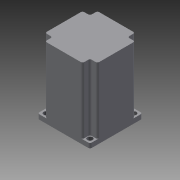
# Autodesk Inventor part: nema23_HS8630
Saved by Autodesk Inventor 2014 (Build 180170000, 170)
## iProperties
Created: 2014-08-18
Part Number: nema23_HS8630
Material: Generic
Document SubType Name: Modeling
Designer: Matthew
Density: 1 g/cm^3
Appearance: Default
Author: Matthew
Autodesk Inventor part; units mm, degrees
ref_plane "YZ Plane" through (0, 0, 0) normal (1, 0, 0) x (0, 1, 0)
ref_plane "XZ Plane" through (0, 0, 0) normal (0, 1, 0) x (-1, 0, 0)
ref_plane "XY Plane" through (0, 0, 0) normal (0, 0, 1) x (1, 0, 0)
sketch "Sketch1" plane through (0, 0, 0) normal (0, 0, 1) x (1, 0, 0)
  line L0 (-28.2, -28.2) -> (28.2, -28.2)
  line L1 (28.2, -28.2) -> (28.2, 28.2)
  line L2 (28.2, 28.2) -> (-28.2, 28.2)
  line L3 (-28.2, 28.2) -> (-28.2, -28.2)
  line L4 (-28.2, -28.2) -> (28.2, 28.2) construction
  line L5 (28.2, -28.2) -> (-28.2, 28.2) construction
  point P0 (0, 0)
  point P1 (-23.57, 23.57)
  point P2 (23.57, 23.57)
  point P3 (23.57, -23.57)
  point P4 (-23.57, -23.57)
  dimension "d0" = 56.4
  dimension "d1" = 56.4
  dimension "d2" = 47.14
  constraints: 12 end point, 4 point on line, 2 horizontal alignment, 2 midpoint, 2 parallel, 2 vertical alignment, 1 horizontal, 1 perpendicular
  measures "d0" distance of L2.end L1.end
  measures "d1" distance of L0.end L1.end
  measures "d2" distance of point (23.57, 23.57) point (-23.57, 23.57)
extrude "Extrusion1" add sketch "Sketch1" along normal blind 76
sketch "Sketch2" plane through (0, 0, 0) normal (0, 0, -1) x (-1, 0, 0)
  point P0 (0, 0)
  point P1 (-23.57, 23.57)
  point P2 (23.57, 23.57)
  point P3 (23.57, -23.57)
  point P4 (-23.57, -23.57)
  dimension "d5" = 47.14
  dimension "d6" = 47.14
  dimension "d8" = 23.57
  dimension "d9" = 23.57
  constraints: 2 horizontal alignment, 2 vertical alignment
  measures "d5" distance of point (23.57, 23.57) point (-23.57, 23.57)
  measures "d6" distance of point (23.57, -23.57) point (23.57, 23.57)
  measures "d8" horizontal distance of point (0, 0) point (-23.57, 23.57)
  measures "d9" horizontal distance of point (-23.57, -23.57) point (0, 0)
hole "Hole1" at (23.57, 23.57, 0) at (-23.57, 23.57, 0) at (-23.57, -23.57, 0) at (23.57, -23.57, 0) direction (0, 0, 1) diameter 5.5 depth 8 tip angle 118
thread "Thread1" size "M5x0.8" class "6H" standard "ANSI Metric M Profile" full length
thread "Thread2" size "M5.5x0.5" class "6H" standard "ANSI Metric M Profile" full length
thread "Thread3" size "M5.5x0.5" class "6H" standard "ANSI Metric M Profile" full length
thread "Thread4" size "M5.5x0.5" class "6H" standard "ANSI Metric M Profile" full length
sketch "Sketch3" plane through (0, 0, 0) normal (0, 0, -1) x (-1, 0, 0)
  circle A0 centre (0, 0) radius 19.05
  dimension "d25" = 38.1
  constraints: 1 centre point, 1 coincident
  measures "d25" diameter of A0
extrude "Extrusion2" add sketch "Sketch3" along normal blind 1.6
sketch "Sketch4" plane through (0, 0, -1.6) normal (0, 0, -1) x (-1, 0, 0)
  circle A0 centre (0, 0) radius 19.05 projected
  circle A1 centre (0, 0) radius 3.175
  dimension "d28" = 6.35
  constraints: 1 centre point, 1 coincident
  measures "d28" diameter of A1
extrude "Extrusion3" add sketch "Sketch4" along normal blind 21 contours A1
sketch "Sketch5" plane through (0, 0, 76) normal (0, 0, 1) x (1, 0, 0)
  line L0 (-28.2, -28.2) -> (28.2, -28.2) projected
  line L1 (28.2, -28.2) -> (28.2, 28.2) projected
  line L2 (28.2, 28.2) -> (-28.2, 28.2) projected
  line L3 (-28.2, 28.2) -> (-28.2, -28.2) projected
  line L4 (-28.2, 20.2) -> (-20.2, 20.2)
  line L5 (-20.2, 20.2) -> (-20.2, 28.2)
  line L6 (20.2, 28.2) -> (20.2, 20.2)
  line L7 (20.2, 20.2) -> (28.2, 20.2)
  line L8 (28.2, -20.2) -> (20.2, -20.2)
  line L9 (-20.2, -28.2) -> (-20.2, -20.2)
  line L10 (-20.2, -20.2) -> (-28.2, -20.2)
  line L11 (20.2, -20.2) -> (20.2, -28.2)
  line L12 (-20.2, 28.2) -> (20.2, 28.2)
  line L13 (28.2, 20.2) -> (28.2, -20.2)
  line L14 (-28.2, 20.2) -> (-28.2, -20.2)
  line L15 (-20.2, -28.2) -> (20.2, -28.2)
  point P0 (0, 0)
  dimension "d31" = 8
  dimension "d32" = 8
  dimension "d33" = 8
  dimension "d34" = 8
  dimension "d35" = 8
  dimension "d36" = 8
  dimension "d37" = 8
  dimension "d38" = 8
  constraints: 24 end point, 8 point on line, 6 perpendicular, 3 collinear, 2 parallel
  measures "d31" distance of L4.start L4.end
  measures "d32" distance of L4.end L5.end
  measures "d33" distance of L9.end L10.end
  measures "d34" distance of L9.start L9.end
  measures "d35" distance of L8.end L11.end
  measures "d36" distance of L8.start L8.end
  measures "d37" distance of L6.end L7.end
  measures "d38" distance of L6.start L6.end
extrude "Extrusion4" cut sketch "Sketch5" against normal blind 71 contours L3 L10 L9 L0 | L11 L8 L1 L0 | L3 L2 L5 L4 | L7 L6 L2 L1
fillet "Fillet1" radius 2 1 edges at (-28.2, 28.2, 2.5)
fillet "Fillet2" radius 2 15 edges at (28.2, 28.2, 2.5) (-20.2, 28.2, 40.5) (-28.2, 20.2, 40.5) (-20.2, 20.2, 40.5) (-28.2, -20.2, 40.5) (-28.2, -28.2, 2.5) (20.2, 28.2, 40.5) (20.2, 20.2, 40.5) (28.2, 20.2, 40.5) (20.2, -28.2, 40.5) (20.2, -20.2, 40.5) (28.2, -20.2, 40.5) (28.2, -28.2, 2.5) (-20.2, -28.2, 40.5) (-20.2, -20.2, 40.5)
equation "\"d1\" = d0"
equation "\"d6\" = d5"
equation "\"d8\" = 0.5 * d5"
equation "\"d9\" = d8"
equation "\"d33\" = d31"
equation "\"d34\" = d32"
equation "\"d35\" = d34"
equation "\"d36\" = d35"
equation "\"d37\" = d31"
equation "\"d38\" = d32"
body "Solid1"
